Autodesk Fusion 360 part; units mm, degrees
(part 3 of 6)
  constraint coincident L336.end L337.start
  constraint perpendicular L693 L694
  constraint parallel L693 L695
  constraint parallel L694 L696
  constraint coincident L473.end L474.start
  constraint perpendicular L473 L693
  constraint coincident L504.end L505.start
  constraint perpendicular L697 L698
  constraint parallel L697 L699
  constraint parallel L698 L700
  constraint perpendicular L701 L702
  constraint parallel L701 L703
  constraint parallel L702 L704
  constraint coincident L458.end L459.start
  constraint perpendicular L458 L701
  constraint coincident L474.end L475.start
  constraint perpendicular L705 L706
  constraint parallel L705 L707
  constraint parallel L706 L708
  constraint perpendicular L709 L710
  constraint parallel L709 L711
  constraint parallel L710 L712
  constraint coincident L429.end L430.start
  constraint perpendicular L429 L709
  constraint coincident L440.start L459.end
  constraint perpendicular L713 L714
  constraint parallel L713 L715
  constraint parallel L714 L716
  constraint perpendicular L717 L718
  constraint parallel L717 L719
  constraint parallel L718 L720
  constraint coincident L385.end L386.start
  constraint perpendicular L385 L717
  constraint coincident L430.end L431.start
  constraint perpendicular L721 L722
  constraint parallel L721 L723
  constraint parallel L722 L724
  constraint coincident L356.end L357.start
  constraint perpendicular L357 L721
  constraint coincident L420.start L439.end
  constraint perpendicular L725 L726
  constraint parallel L725 L727
  constraint parallel L726 L728
  constraint coincident L386.end L387.start
  constraint perpendicular L387 L725
  constraint coincident L410.end L411.start
  constraint perpendicular L729 L730
  constraint parallel L729 L731
  constraint parallel L730 L732
  constraint coincident L401.end L402.start
  constraint perpendicular L402 L729
  constraint coincident L355.end L356.start
  constraint perpendicular L733 L734
  constraint parallel L733 L735
  constraint parallel L734 L736
  constraint coincident L484.end L485.start
  constraint perpendicular L485 L733
  constraint coincident L400.end L401.start
  constraint perpendicular L737 L738
  constraint parallel L737 L739
  constraint parallel L738 L740
  constraint coincident L493.end L494.start
  constraint perpendicular L493 L737
  constraint coincident L411.end L412.start
  constraint perpendicular L741 L742
  constraint parallel L741 L743
  constraint parallel L742 L744
  constraint coincident L326.end L327.start
  constraint perpendicular L326 L741
  constraint coincident L494.end L495.start
  constraint perpendicular L745 L746
  constraint parallel L745 L747
  constraint parallel L746 L748
  constraint coincident L337.end L338.start
  constraint perpendicular L338 L745
  constraint coincident L483.end L484.start
  constraint perpendicular L749 L750
  constraint parallel L749 L751
  constraint parallel L750 L752
  constraint coincident L127.end L128.start
  constraint perpendicular L127 L749
  constraint coincident L586.end L587.start
  constraint perpendicular L753 L754
  constraint parallel L753 L755
  constraint parallel L754 L756
  constraint coincident L595.end L596.start
  constraint perpendicular L595 L753
  constraint coincident L138.end L139.start
  constraint perpendicular L757 L758
  constraint parallel L757 L759
  constraint parallel L758 L760
  constraint coincident L294.end L295.start
  constraint perpendicular L295 L757
  constraint coincident L81.end L82.start
  constraint perpendicular L761 L762
  constraint parallel L761 L763
  constraint parallel L762 L764
  constraint coincident L92.end L93.start
  constraint perpendicular L93 L761
  constraint coincident L283.end L284.start
  constraint perpendicular L765 L766
  constraint parallel L765 L767
  constraint parallel L766 L768
  constraint coincident L197.end L198.start
  constraint perpendicular L198 L765
  constraint coincident L91.end L92.start
  constraint perpendicular L769 L770
  constraint parallel L769 L771
  constraint parallel L770 L772
  constraint perpendicular L773 L774
  constraint parallel L773 L775
  constraint parallel L774 L776
  constraint coincident L545.end L546.start
  constraint perpendicular L546 L773
  constraint coincident L571.end L572.start
  constraint perpendicular L777 L778
  constraint parallel L777 L779
  constraint parallel L778 L780
  constraint perpendicular L781 L782
  constraint parallel L781 L783
  constraint parallel L782 L784
  constraint coincident L151.end L152.start
  constraint perpendicular L152 L781
  constraint coincident L162.end L163.start
  constraint perpendicular L785 L786
  constraint parallel L785 L787
  constraint parallel L786 L788
  constraint perpendicular L789 L790
  constraint parallel L789 L791
  constraint parallel L790 L792
  constraint coincident L28.end L29.start
  constraint perpendicular L28 L789
  constraint coincident L536.end L537.start
  constraint perpendicular L793 L794
  constraint parallel L793 L795
  constraint parallel L794 L796
  constraint perpendicular L797 L798
  constraint parallel L797 L799
  constraint parallel L798 L800
  constraint coincident L232.end L233.start
  constraint perpendicular L233 L797
  constraint coincident L213.end L214.start
  constraint perpendicular L801 L802
  constraint parallel L801 L803
  constraint parallel L802 L804
  constraint perpendicular L805 L806
  constraint parallel L805 L807
  constraint parallel L806 L808
  constraint coincident L70.end L71.start
  constraint perpendicular L70 L805
  constraint coincident L51.end L52.start
  constraint perpendicular L809 L810
  constraint parallel L809 L811
  constraint parallel L810 L812
  constraint perpendicular L813 L814
  constraint parallel L813 L815
  constraint parallel L814 L816
  constraint coincident L277.end L278.start
  constraint perpendicular L278 L813
  constraint coincident L240.start L259.end
  constraint perpendicular L817 L818
  constraint parallel L817 L819
  constraint parallel L818 L820
  constraint perpendicular L821 L822
  constraint parallel L821 L823
  constraint parallel L822 L824
  constraint coincident L107.end L108.start
  constraint perpendicular L107 L821
  constraint coincident L17.end L18.start
  constraint perpendicular L825 L826
  constraint parallel L825 L827
  constraint parallel L826 L828
  constraint perpendicular L829 L830
  constraint parallel L829 L831
  constraint parallel L830 L832
  constraint coincident L284.end L285.start
  constraint perpendicular L285 L829
  constraint coincident L317.end L318.start
  constraint perpendicular L833 L834
  constraint parallel L833 L835
  constraint parallel L834 L836
  measures "d21" distance of L503.end L687.end
  measures "d22" distance of L336.end L691.end
  measures "d23" distance of L586.end L751.end
  measures "d24" distance of L138.end L755.end
  measures "d25" distance of L81.end L759.end
  measures "d26" distance of L283.end L763.end
extrude "Extrude4" cut sketch "Sketch3" against normal blind 20 contours L17 L753 L755 L820 L824 L826 | L108 L753 L755 L822 L828 L834 | L71 L753 L755 L806 L812 L818 | L7 L749 L751 L820 L826 | L138 L753 L755 L756 L836 | L118 L749 L751 L828 L834 | L51 L753 L755 L804 L808 L810 | L61 L749 L751 L812 L818 | L267 L757 L759 L820 L826 | L128 L749 L750 L751 L836 | L308 L757 L759 L828 L834 | L29 L753 L755 L790 L796 L802 | L41 L749 L751 L804 L810 | L250 L757 L759 L812 L818 | L294 L757 L758 L759 L836 | L536 L753 L755 L788 L792 L794 | L39 L749 L751 L796 L802 | L222 L757 L759 L804 L810 | L572 L753 L755 L776 L778 L786 | L526 L749 L751 L788 L794 | L204 L757 L759 L796 L802 | L277 L761 L763 L814 L820 L826 | L318 L761 L763 L828 L832 L834 | L545 L753 L755 L772 L774 L780 | L562 L749 L751 L778 L786 | L141 L757 L759 L788 L794 | L240 L761 L763 L812 L816 L818 | L284 L761 L763 L764 L830 L836 | L596 L753 L754 L755 L770 | L555 L749 L751 L772 L780 | L173 L757 L759 L778 L786 | L232 L761 L763 L798 L804 L810 | L586 L749 L751 L752 L770 | L187 L757 L759 L772 L780 | L214 L761 L763 L796 L800 L802 | L82 L757 L759 L760 L770 | L151 L761 L763 L782 L788 L794 | L163 L761 L763 L778 L784 L786 | L197 L761 L763 L766 L772 L780 | L92 L761 L762 L763 L768 L770 | L337 L689 L691 L692 L746 | L484 L689 L691 L734 L748 | L401 L689 L691 L730 L736 | L327 L685 L686 L687 L742 | L494 L685 L687 L738 L744 | L356 L689 L691 L722 L732 | L411 L685 L687 L728 L740 | L420 L689 L691 L714 L724 | L386 L685 L687 L718 L726 | L449 L689 L691 L708 L716 | L430 L685 L687 L710 L714 L720 | L464 L689 L691 L698 L706 | L459 L685 L687 L702 L708 L712 L716 | L514 L689 L690 L691 L700 | L474 L685 L687 L694 L698 L704 L706 | L504 L685 L687 L688 L696 L700
extrude "Extrude6" add sketch "Sketch3" against normal blind 1 contours L17 L753 L755 L820 L824 L826 | L108 L753 L755 L822 L828 L834 | L71 L753 L755 L806 L812 L818 | L7 L749 L751 L820 L826 | L138 L753 L755 L756 L836 | L118 L749 L751 L828 L834 | L51 L753 L755 L804 L808 L810 | L61 L749 L751 L812 L818 | L267 L757 L759 L820 L826 | L128 L749 L750 L751 L836 | L308 L757 L759 L828 L834 | L29 L753 L755 L790 L796 L802 | L41 L749 L751 L804 L810 | L250 L757 L759 L812 L818 | L294 L757 L758 L759 L836 | L536 L753 L755 L788 L792 L794 | L39 L749 L751 L796 L802 | L222 L757 L759 L804 L810 | L572 L753 L755 L776 L778 L786 | L526 L749 L751 L788 L794 | L204 L757 L759 L796 L802 | L277 L761 L763 L814 L820 L826 | L318 L761 L763 L828 L832 L834 | L545 L753 L755 L772 L774 L780 | L562 L749 L751 L778 L786 | L141 L757 L759 L788 L794 | L240 L761 L763 L812 L816 L818 | L284 L761 L763 L764 L830 L836 | L596 L753 L754 L755 L770 | L555 L749 L751 L772 L780 | L173 L757 L759 L778 L786 | L232 L761 L763 L798 L804 L810 | L586 L749 L751 L752 L770 | L187 L757 L759 L772 L780 | L214 L761 L763 L796 L800 L802 | L82 L757 L759 L760 L770 | L151 L761 L763 L782 L788 L794 | L163 L761 L763 L778 L784 L786 | L197 L761 L763 L766 L772 L780 | L92 L761 L762 L763 L768 L770 | L337 L689 L691 L692 L746 | L484 L689 L691 L734 L748 | L401 L689 L691 L730 L736 | L327 L685 L686 L687 L742 | L494 L685 L687 L738 L744 | L356 L689 L691 L722 L732 | L411 L685 L687 L728 L740 | L420 L689 L691 L714 L724 | L386 L685 L687 L718 L726 | L449 L689 L691 L708 L716 | L430 L685 L687 L710 L714 L720 | L464 L689 L691 L698 L706 | L459 L685 L687 L702 L708 L712 L716 | L514 L689 L690 L691 L700 | L474 L685 L687 L694 L698 L704 L706 | L504 L685 L687 L688 L696 L700
sketch "Sketch4" plane through (0, -4, 0) normal (0, -1, 0) x (1, 0, 0)
  line L0 (39.9203, -25.9319) -> (39.9203, -22.8327)
  line L1 (39.9203, -22.8327) -> (40.7211, -22.8327)
  line L2 (40.7211, -22.8327) -> (40.7211, -20.8323)
  line L3 (54.7204, -20.8323) -> (54.7204, -22.8327)
  line L4 (54.7204, -22.8327) -> (55.5212, -22.8327)
  line L5 (55.5212, -22.8327) -> (55.5212, -25.9319)
  line L6 (55.5212, -25.9319) -> (54.7204, -25.9319)
  line L7 (54.7204, -25.9319) -> (54.7204, -31.7321)
  line L8 (54.7204, -31.7321) -> (55.5212, -31.7321)
  line L9 (55.5212, -31.7321) -> (55.5212, -34.8327)
  line L10 (55.5212, -34.8327) -> (54.7204, -34.8327)
  line L11 (54.7204, -34.8327) -> (54.7204, -36.8316)
  line L12 (40.7211, -36.8316) -> (40.7211, -34.8327)
  line L13 (40.7211, -34.8327) -> (39.9203, -34.8327)
  line L14 (39.9203, -34.8327) -> (39.9203, -31.7321)
  line L15 (39.9203, -31.7321) -> (40.7211, -31.7321)
  line L16 (40.7211, -31.7321) -> (40.7211, -25.9319)
  line L17 (40.7211, -25.9319) -> (39.9203, -25.9319)
  line L18 (111.869, -34.8327) -> (111.869, -36.8316)
  line L19 (97.8697, -36.8316) -> (97.8697, -34.8327)
  line L20 (97.8697, -34.8327) -> (97.0703, -34.8327)
  line L21 (97.0703, -34.8327) -> (97.0703, -31.7321)
  line L22 (97.0703, -31.7321) -> (97.8697, -31.7321)
  line L23 (97.8697, -31.7321) -> (97.8697, -25.9319)
  line L24 (97.8697, -25.9319) -> (97.0703, -25.9319)
  line L25 (97.0703, -25.9319) -> (97.0703, -22.8327)
  line L26 (97.0703, -22.8327) -> (97.8697, -22.8327)
  line L27 (97.8697, -22.8327) -> (97.8697, -20.8323)
  line L28 (111.869, -20.8323) -> (111.869, -22.8327)
  line L29 (111.869, -22.8327) -> (112.67, -22.8327)
  line L30 (112.67, -22.8327) -> (112.67, -25.9319)
  line L31 (112.67, -25.9319) -> (111.869, -25.9319)
  line L32 (111.869, -25.9319) -> (111.869, -31.7321)
  line L33 (111.869, -31.7321) -> (112.67, -31.7321)
  line L34 (112.67, -31.7321) -> (112.67, -34.8327)
  line L35 (112.67, -34.8327) -> (111.869, -34.8327)
  line L36 (78.8211, -36.8316) -> (78.8211, -34.8327)
  line L37 (78.8211, -34.8327) -> (78.0203, -34.8327)
  line L38 (78.0203, -34.8327) -> (78.0203, -31.7321)
  line L39 (78.0203, -31.7321) -> (78.8211, -31.7321)
  line L40 (78.8211, -31.7321) -> (78.8211, -25.9319)
  line L41 (78.8211, -25.9319) -> (78.0203, -25.9319)
  line L42 (78.0203, -25.9319) -> (78.0203, -22.8327)
  line L43 (78.0203, -22.8327) -> (78.8211, -22.8327)
  line L44 (78.8211, -22.8327) -> (78.8211, -20.8323)
  line L45 (92.8204, -20.8323) -> (92.8204, -22.8327)
  line L46 (92.8204, -22.8327) -> (93.6198, -22.8327)
  line L47 (93.6198, -22.8327) -> (93.6198, -25.9319)
  line L48 (93.6198, -25.9319) -> (92.8204, -25.9319)
  line L49 (92.8204, -25.9319) -> (92.8204, -31.7321)
  line L50 (92.8204, -31.7321) -> (93.6198, -31.7321)
  line L51 (93.6198, -31.7321) -> (93.6198, -34.8327)
  line L52 (93.6198, -34.8327) -> (92.8204, -34.8327)
  line L53 (92.8204, -34.8327) -> (92.8204, -36.8316)
  line L54 (59.7711, -36.8316) -> (59.7711, -34.8327)
  line L55 (59.7711, -34.8327) -> (58.9703, -34.8327)
  line L56 (58.9703, -34.8327) -> (58.9703, -31.7321)
  line L57 (58.9703, -31.7321) -> (59.7711, -31.7321)
  line L58 (59.7711, -31.7321) -> (59.7711, -25.9319)
  line L59 (59.7711, -25.9319) -> (58.9703, -25.9319)
  line L60 (58.9703, -25.9319) -> (58.9703, -22.8327)
  line L61 (58.9703, -22.8327) -> (59.7711, -22.8327)
  line L62 (59.7711, -22.8327) -> (59.7711, -20.8323)
  line L63 (73.7704, -20.8323) -> (73.7704, -22.8327)
  line L64 (73.7704, -22.8327) -> (74.5712, -22.8327)
  line L65 (74.5712, -22.8327) -> (74.5712, -25.9319)
  line L66 (74.5712, -25.9319) -> (73.7704, -25.9319)
  line L67 (73.7704, -25.9319) -> (73.7704, -31.7321)
  line L68 (73.7704, -31.7321) -> (74.5712, -31.7321)
  line L69 (74.5712, -31.7321) -> (74.5712, -34.8327)
  line L70 (74.5712, -34.8327) -> (73.7704, -34.8327)
  line L71 (73.7704, -34.8327) -> (73.7704, -36.8316)
  line L72 (188.07, -41.8828) -> (188.871, -41.8828)
  line L73 (188.871, -41.8828) -> (188.871, -44.982)
  line L74 (188.871, -44.982) -> (188.07, -44.982)
  line L75 (188.07, -44.982) -> (188.07, -50.782)
  line L76 (188.07, -50.782) -> (188.871, -50.782)
  line L77 (188.871, -50.782) -> (188.871, -53.8826)
  line L78 (188.871, -53.8826) -> (188.07, -53.8826)
  line L79 (188.07, -53.8826) -> (188.07, -55.8816)
  line L80 (174.071, -55.8816) -> (174.071, -53.8826)
  line L81 (174.071, -53.8826) -> (173.27, -53.8826)
  line L82 (173.27, -53.8826) -> (173.27, -50.782)
  line L83 (173.27, -50.782) -> (174.071, -50.782)
  line L84 (174.071, -50.782) -> (174.071, -44.982)
  line L85 (174.071, -44.982) -> (173.27, -44.982)
  line L86 (173.27, -44.982) -> (173.27, -41.8828)
  line L87 (173.27, -41.8828) -> (174.071, -41.8828)
  line L88 (174.071, -41.8828) -> (174.071, -39.8824)
  line L89 (188.07, -39.8824) -> (188.07, -41.8828)
  line L90 (36.4712, -34.8327) -> (35.6704, -34.8327)
  line L91 (35.6704, -34.8327) -> (35.6704, -36.8316)
  line L92 (21.671, -36.8316) -> (21.671, -34.8327)
  line L93 (21.671, -34.8327) -> (20.8704, -34.8327)
  line L94 (20.8704, -34.8327) -> (20.8704, -31.7321)
  line L95 (20.8704, -31.7321) -> (21.671, -31.7321)
  line L96 (21.671, -31.7321) -> (21.671, -25.9319)
  line L97 (21.671, -25.9319) -> (20.8704, -25.9319)
  line L98 (20.8704, -25.9319) -> (20.8704, -22.8327)
  line L99 (20.8704, -22.8327) -> (21.671, -22.8327)
  line L100 (21.671, -22.8327) -> (21.671, -20.8323)
  line L101 (35.6704, -20.8323) -> (35.6704, -22.8327)
  line L102 (35.6704, -22.8327) -> (36.4712, -22.8327)
  line L103 (36.4712, -22.8327) -> (36.4712, -25.9319)
  line L104 (36.4712, -25.9319) -> (35.6704, -25.9319)
  line L105 (35.6704, -25.9319) -> (35.6704, -31.7321)
  line L106 (35.6704, -31.7321) -> (36.4712, -31.7321)
  line L107 (36.4712, -31.7321) -> (36.4712, -34.8327)
  line L108 (1.8204, -22.8327) -> (2.621, -22.8327)
  line L109 (2.621, -22.8327) -> (2.621, -20.8323)
  line L110 (16.6205, -20.8323) -> (16.6205, -22.8327)
  line L111 (16.6205, -22.8327) -> (17.4212, -22.8327)
  line L112 (17.4212, -22.8327) -> (17.4212, -25.9319)
  line L113 (17.4212, -25.9319) -> (16.6205, -25.9319)
  line L114 (16.6205, -25.9319) -> (16.6205, -31.7321)
  line L115 (16.6205, -31.7321) -> (17.4212, -31.7321)
  line L116 (17.4212, -31.7321) -> (17.4212, -34.8327)
  line L117 (17.4212, -34.8327) -> (16.6205, -34.8327)
  line L118 (16.6205, -34.8327) -> (16.6205, -36.8316)
  line L119 (2.621, -36.8316) -> (2.621, -34.8327)
  line L120 (2.621, -34.8327) -> (1.8204, -34.8327)
  line L121 (1.8204, -34.8327) -> (1.8204, -31.7321)
  line L122 (1.8204, -31.7321) -> (2.621, -31.7321)
  line L123 (2.621, -31.7321) -> (2.621, -25.9319)
  line L124 (2.621, -25.9319) -> (1.8204, -25.9319)
  line L125 (1.8204, -25.9319) -> (1.8204, -22.8327)
  line L126 (130.92, -39.8824) -> (130.92, -41.8828)
  line L127 (130.92, -41.8828) -> (131.721, -41.8828)
  line L128 (131.721, -41.8828) -> (131.721, -44.982)
  line L129 (131.721, -44.982) -> (130.92, -44.982)
  line L130 (130.92, -44.982) -> (130.92, -50.782)
  line L131 (130.92, -50.782) -> (131.721, -50.782)
  line L132 (131.721, -50.782) -> (131.721, -53.8826)
  line L133 (131.721, -53.8826) -> (130.92, -53.8826)
  line L134 (130.92, -53.8826) -> (130.92, -55.8816)
  line L135 (116.92, -55.8816) -> (116.92, -53.8826)
  line L136 (116.92, -53.8826) -> (116.119, -53.8826)
  line L137 (116.119, -53.8826) -> (116.119, -50.782)
  line L138 (116.119, -50.782) -> (116.92, -50.782)
  line L139 (116.92, -50.782) -> (116.92, -44.982)
  line L140 (116.92, -44.982) -> (116.119, -44.982)
  line L141 (116.119, -44.982) -> (116.119, -41.8828)
  line L142 (116.119, -41.8828) -> (116.92, -41.8828)
  line L143 (116.92, -41.8828) -> (116.92, -39.8824)
  line L144 (135.17, -53.8826) -> (135.17, -50.782)
  line L145 (135.17, -50.782) -> (135.971, -50.782)
  line L146 (135.971, -50.782) -> (135.971, -44.982)
  line L147 (135.971, -44.982) -> (135.17, -44.982)
  line L148 (135.17, -44.982) -> (135.17, -41.8828)
  line L149 (135.17, -41.8828) -> (135.971, -41.8828)
  line L150 (135.971, -41.8828) -> (135.971, -39.8824)
  line L151 (149.97, -39.8824) -> (149.97, -41.8828)
  line L152 (149.97, -41.8828) -> (150.771, -41.8828)
  line L153 (150.771, -41.8828) -> (150.771, -44.982)
  line L154 (150.771, -44.982) -> (149.97, -44.982)
  line L155 (149.97, -44.982) -> (149.97, -50.782)
  line L156 (149.97, -50.782) -> (150.771, -50.782)
  line L157 (150.771, -50.782) -> (150.771, -53.8826)
  line L158 (150.771, -53.8826) -> (149.97, -53.8826)
  line L159 (149.97, -53.8826) -> (149.97, -55.8816)
  line L160 (135.971, -55.8816) -> (135.971, -53.8826)
  line L161 (135.971, -53.8826) -> (135.17, -53.8826)
  line L162 (169.821, -50.782) -> (169.821, -53.8826)
  line L163 (169.821, -53.8826) -> (169.02, -53.8826)
  line L164 (169.02, -53.8826) -> (169.02, -55.8816)
  line L165 (155.021, -55.8816) -> (155.021, -53.8826)
  line L166 (155.021, -53.8826) -> (154.22, -53.8826)
  line L167 (154.22, -53.8826) -> (154.22, -50.782)
  line L168 (154.22, -50.782) -> (155.021, -50.782)
  line L169 (155.021, -50.782) -> (155.021, -44.982)
  line L170 (155.021, -44.982) -> (154.22, -44.982)
  line L171 (154.22, -44.982) -> (154.22, -41.8828)
  line L172 (154.22, -41.8828) -> (155.021, -41.8828)
  line L173 (155.021, -41.8828) -> (155.021, -39.8824)
  line L174 (169.02, -39.8824) -> (169.02, -41.8828)
  line L175 (169.02, -41.8828) -> (169.821, -41.8828)
  line L176 (169.821, -41.8828) -> (169.821, -44.982)
  line L177 (169.821, -44.982) -> (169.02, -44.982)
  line L178 (169.02, -44.982) -> (169.02, -50.782)
  line L179 (169.02, -50.782) -> (169.821, -50.782)
  line L180 (112.67, -44.982) -> (111.869, -44.982)
  line L181 (111.869, -44.982) -> (111.869, -50.782)
  line L182 (111.869, -50.782) -> (112.67, -50.782)
  line L183 (112.67, -50.782) -> (112.67, -53.8826)
  line L184 (112.67, -53.8826) -> (111.869, -53.8826)
  line L185 (111.869, -53.8826) -> (111.869, -55.8816)
  line L186 (97.8697, -55.8816) -> (97.8697, -53.8826)
  line L187 (97.8697, -53.8826) -> (97.0703, -53.8826)
  line L188 (97.0703, -53.8826) -> (97.0703, -50.782)
  line L189 (97.0703, -50.782) -> (97.8697, -50.782)
  line L190 (97.8697, -50.782) -> (97.8697, -44.982)
  line L191 (97.8697, -44.982) -> (97.0703, -44.982)
  line L192 (97.0703, -44.982) -> (97.0703, -41.8828)
  line L193 (97.0703, -41.8828) -> (97.8697, -41.8828)
  line L194 (97.8697, -41.8828) -> (97.8697, -39.8824)
  line L195 (111.869, -39.8824) -> (111.869, -41.8828)
  line L196 (111.869, -41.8828) -> (112.67, -41.8828)
  line L197 (112.67, -41.8828) -> (112.67, -44.982)
  line L198 (92.8204, -41.8828) -> (93.6198, -41.8828)
  line L199 (93.6198, -41.8828) -> (93.6198, -44.982)
  line L200 (93.6198, -44.982) -> (92.8204, -44.982)
  line L201 (92.8204, -44.982) -> (92.8204, -50.782)
  line L202 (92.8204, -50.782) -> (93.6198, -50.782)
  line L203 (93.6198, -50.782) -> (93.6198, -53.8826)
  line L204 (93.6198, -53.8826) -> (92.8204, -53.8826)
  line L205 (92.8204, -53.8826) -> (92.8204, -55.8816)
  line L206 (78.8211, -55.8816) -> (78.8211, -53.8826)
  line L207 (78.8211, -53.8826) -> (78.0203, -53.8826)
  line L208 (78.0203, -53.8826) -> (78.0203, -50.782)
  line L209 (78.0203, -50.782) -> (78.8211, -50.782)
  line L210 (78.8211, -50.782) -> (78.8211, -44.982)
  line L211 (78.8211, -44.982) -> (78.0203, -44.982)
  line L212 (78.0203, -44.982) -> (78.0203, -41.8828)
  line L213 (78.0203, -41.8828) -> (78.8211, -41.8828)
  line L214 (78.8211, -41.8828) -> (78.8211, -39.8824)
  line L215 (92.8204, -39.8824) -> (92.8204, -41.8828)
  line L216 (59.7711, -55.8816) -> (59.7711, -53.8826)
  line L217 (59.7711, -53.8826) -> (58.9703, -53.8826)
  line L218 (58.9703, -53.8826) -> (58.9703, -50.782)
  line L219 (58.9703, -50.782) -> (59.7711, -50.782)
  line L220 (59.7711, -50.782) -> (59.7711, -44.982)
  line L221 (59.7711, -44.982) -> (58.9703, -44.982)
  line L222 (58.9703, -44.982) -> (58.9703, -41.8828)
  line L223 (58.9703, -41.8828) -> (59.7711, -41.8828)
  line L224 (59.7711, -41.8828) -> (59.7711, -39.8824)
  line L225 (73.7704, -39.8824) -> (73.7704, -41.8828)
  line L226 (73.7704, -41.8828) -> (74.5712, -41.8828)
  line L227 (74.5712, -41.8828) -> (74.5712, -44.982)
  line L228 (74.5712, -44.982) -> (73.7704, -44.982)
  line L229 (73.7704, -44.982) -> (73.7704, -50.782)
  line L230 (73.7704, -50.782) -> (74.5712, -50.782)
  line L231 (74.5712, -50.782) -> (74.5712, -53.8826)
  line L232 (74.5712, -53.8826) -> (73.7704, -53.8826)
  line L233 (73.7704, -53.8826) -> (73.7704, -55.8816)
  line L234 (55.5212, -50.782) -> (55.5212, -53.8826)
  line L235 (55.5212, -53.8826) -> (54.7204, -53.8826)
  line L236 (54.7204, -53.8826) -> (54.7204, -55.8816)
  line L237 (40.7211, -55.8816) -> (40.7211, -53.8826)
  line L238 (40.7211, -53.8826) -> (39.9203, -53.8826)
  line L239 (39.9203, -53.8826) -> (39.9203, -50.782)
  line L240 (39.9203, -50.782) -> (40.7211, -50.782)
  line L241 (40.7211, -50.782) -> (40.7211, -44.982)
  line L242 (40.7211, -44.982) -> (39.9203, -44.982)
  line L243 (39.9203, -44.982) -> (39.9203, -41.8828)
  line L244 (39.9203, -41.8828) -> (40.7211, -41.8828)
  line L245 (40.7211, -41.8828) -> (40.7211, -39.8824)
  line L246 (54.7204, -39.8824) -> (54.7204, -41.8828)
  line L247 (54.7204, -41.8828) -> (55.5212, -41.8828)
  line L248 (55.5212, -41.8828) -> (55.5212, -44.982)
  line L249 (55.5212, -44.982) -> (54.7204, -44.982)
  line L250 (54.7204, -44.982) -> (54.7204, -50.782)
  line L251 (54.7204, -50.782) -> (55.5212, -50.782)
  line L252 (1.8204, -50.782) -> (2.621, -50.782)
  line L253 (2.621, -50.782) -> (2.621, -44.982)
  line L254 (2.621, -44.982) -> (1.8204, -44.982)
  line L255 (1.8204, -44.982) -> (1.8204, -41.8828)
  line L256 (1.8204, -41.8828) -> (2.621, -41.8828)
  line L257 (2.621, -41.8828) -> (2.621, -39.8824)
  line L258 (16.6205, -39.8824) -> (16.6205, -41.8828)
  line L259 (16.6205, -41.8828) -> (17.4212, -41.8828)
  line L260 (17.4212, -41.8828) -> (17.4212, -44.982)
  line L261 (17.4212, -44.982) -> (16.6205, -44.982)
  line L262 (16.6205, -44.982) -> (16.6205, -50.782)
  line L263 (16.6205, -50.782) -> (17.4212, -50.782)
  line L264 (17.4212, -50.782) -> (17.4212, -53.8826)
  line L265 (17.4212, -53.8826) -> (16.6205, -53.8826)
  line L266 (16.6205, -53.8826) -> (16.6205, -55.8816)
  line L267 (2.621, -55.8816) -> (2.621, -53.8826)
  line L268 (2.621, -53.8826) -> (1.8204, -53.8826)
  line L269 (1.8204, -53.8826) -> (1.8204, -50.782)
  line L270 (36.4712, -53.8826) -> (35.6704, -53.8826)
  line L271 (35.6704, -53.8826) -> (35.6704, -55.8816)
  line L272 (21.671, -55.8816) -> (21.671, -53.8826)
  line L273 (21.671, -53.8826) -> (20.8704, -53.8826)
  line L274 (20.8704, -53.8826) -> (20.8704, -50.782)
  line L275 (20.8704, -50.782) -> (21.671, -50.782)
  line L276 (21.671, -50.782) -> (21.671, -44.982)
  line L277 (21.671, -44.982) -> (20.8704, -44.982)
  line L278 (20.8704, -44.982) -> (20.8704, -41.8828)
  line L279 (20.8704, -41.8828) -> (21.671, -41.8828)
  line L280 (21.671, -41.8828) -> (21.671, -39.8824)
  line L281 (35.6704, -39.8824) -> (35.6704, -41.8828)
  line L282 (35.6704, -41.8828) -> (36.4712, -41.8828)
  line L283 (36.4712, -41.8828) -> (36.4712, -44.982)
  line L284 (36.4712, -44.982) -> (35.6704, -44.982)
  line L285 (35.6704, -44.982) -> (35.6704, -50.782)
  line L286 (35.6704, -50.782) -> (36.4712, -50.782)
  line L287 (36.4712, -50.782) -> (36.4712, -53.8826)
  line L288 (163.745, -6.8819) -> (163.745, -3.7827)
  line L289 (163.745, -3.7827) -> (164.546, -3.7827)
  line L290 (164.546, -3.7827) -> (164.546, -1.7823)
  line L291 (178.545, -1.7823) -> (178.545, -3.7827)
  line L292 (178.545, -3.7827) -> (179.346, -3.7827)
  line L293 (179.346, -3.7827) -> (179.346, -6.8819)
  line L294 (179.346, -6.8819) -> (178.545, -6.8819)
  line L295 (178.545, -6.8819) -> (178.545, -12.6821)
  line L296 (178.545, -12.6821) -> (179.346, -12.6821)
  line L297 (179.346, -12.6821) -> (179.346, -15.7827)
  line L298 (179.346, -15.7827) -> (178.545, -15.7827)
  line L299 (178.545, -15.7827) -> (178.545, -17.7817)
  line L300 (164.546, -17.7817) -> (164.546, -15.7827)
  line L301 (164.546, -15.7827) -> (163.745, -15.7827)
  line L302 (163.745, -15.7827) -> (163.745, -12.6821)
  line L303 (163.745, -12.6821) -> (164.546, -12.6821)
  line L304 (164.546, -12.6821) -> (164.546, -6.8819)
  line L305 (164.546, -6.8819) -> (163.745, -6.8819)
  line L306 (120.971, -12.0826) -> (120.146, -12.0826)
  line L307 (120.146, -12.0826) -> (120.146, -15.3128)
  line L308 (120.146, -15.3128) -> (118.42, -15.3128)
  line L309 (118.42, -15.3128) -> (118.42, -16.2319)
  line L310 (118.42, -16.2319) -> (115.12, -16.2319)
  line L311 (115.12, -16.2319) -> (115.12, -15.3128)
  line L312 (115.12, -15.3128) -> (113.396, -15.3128)
  line L313 (113.396, -15.3128) -> (113.396, -12.0826)
  line L314 (113.396, -12.0826) -> (111.87, -12.0826)
  line L315 (111.87, -12.0826) -> (111.87, -12.6821)
  line L316 (111.87, -12.6821) -> (112.671, -12.6821)
  line L317 (112.671, -12.6821) -> (112.671, -15.7827)
  line L318 (112.671, -15.7827) -> (111.87, -15.7827)
  line L319 (111.87, -15.7827) -> (111.87, -17.7817)
  line L320 (97.8711, -17.7817) -> (97.8711, -15.7827)
  line L321 (97.8711, -15.7827) -> (97.0703, -15.7827)
  line L322 (97.0703, -15.7827) -> (97.0703, -12.6821)
  line L323 (97.0703, -12.6821) -> (97.8711, -12.6821)
  line L324 (97.8711, -12.6821) -> (97.8711, -12.0826)
  line L325 (97.8711, -12.0826) -> (96.3454, -12.0826)
  line L326 (96.3454, -12.0826) -> (96.3454, -15.3128)
  line L327 (96.3454, -15.3128) -> (94.6203, -15.3128)
  line L328 (94.6203, -15.3128) -> (94.6203, -16.2319)
  line L329 (94.6203, -16.2319) -> (91.3197, -16.2319)
  line L330 (91.3197, -16.2319) -> (91.3197, -15.3128)
  line L331 (91.3197, -15.3128) -> (89.596, -15.3128)
  line L332 (89.596, -15.3128) -> (89.596, -12.0826)
  line L333 (89.596, -12.0826) -> (88.7705, -12.0826)
  line L334 (88.7705, -12.0826) -> (88.7705, -9.2825)
  line L335 (88.7705, -9.2825) -> (89.596, -9.2825)
  line L336 (89.596, -9.2825) -> (89.596, -3.0138)
  line L337 (89.596, -3.0138) -> (91.3197, -3.0138)
  line L338 (91.3197, -3.0138) -> (91.3197, -2.0326)
  line L339 (91.3197, -2.0326) -> (94.6203, -2.0326)
  line L340 (94.6203, -2.0326) -> (94.6203, -3.0138)
  line L341 (94.6203, -3.0138) -> (96.3454, -3.0138)
  line L342 (96.3454, -3.0138) -> (96.3454, -7.4827)
  line L343 (96.3454, -7.4827) -> (97.8711, -7.4827)
  line L344 (97.8711, -7.4827) -> (97.8711, -6.8819)
  line L345 (97.8711, -6.8819) -> (97.0703, -6.8819)
  line L346 (97.0703, -6.8819) -> (97.0703, -3.7827)
  line L347 (97.0703, -3.7827) -> (97.8711, -3.7827)
  line L348 (97.8711, -3.7827) -> (97.8711, -1.7823)
  line L349 (111.87, -1.7823) -> (111.87, -3.7827)
  line L350 (111.87, -3.7827) -> (112.671, -3.7827)
  line L351 (112.671, -3.7827) -> (112.671, -6.8819)
  line L352 (112.671, -6.8819) -> (111.87, -6.8819)
  line L353 (111.87, -6.8819) -> (111.87, -7.4827)
  line L354 (111.87, -7.4827) -> (113.396, -7.4827)
  line L355 (113.396, -7.4827) -> (113.396, -3.0138)
  line L356 (113.396, -3.0138) -> (115.12, -3.0138)
  line L357 (115.12, -3.0138) -> (115.12, -2.0326)
  line L358 (115.12, -2.0326) -> (118.42, -2.0326)
  line L359 (118.42, -2.0326) -> (118.42, -3.0138)
  line L360 (118.42, -3.0138) -> (120.146, -3.0138)
  line L361 (120.146, -3.0138) -> (120.146, -9.2825)
  line L362 (120.146, -9.2825) -> (120.971, -9.2825)
  line L363 (120.971, -9.2825) -> (120.971, -12.0826)
  line L364 (140.445, -1.7823) -> (140.445, -3.7827)
  line L365 (140.445, -3.7827) -> (141.246, -3.7827)
  line L366 (141.246, -3.7827) -> (141.246, -6.8819)
  line L367 (141.246, -6.8819) -> (140.445, -6.8819)
  line L368 (140.445, -6.8819) -> (140.445, -12.6821)
  line L369 (140.445, -12.6821) -> (141.246, -12.6821)
  line L370 (141.246, -12.6821) -> (141.246, -15.7827)
  line L371 (141.246, -15.7827) -> (140.445, -15.7827)
  line L372 (140.445, -15.7827) -> (140.445, -17.7817)
  line L373 (126.446, -17.7817) -> (126.446, -15.7827)
  line L374 (126.446, -15.7827) -> (125.645, -15.7827)
  line L375 (125.645, -15.7827) -> (125.645, -12.6821)
  line L376 (125.645, -12.6821) -> (126.446, -12.6821)
  line L377 (126.446, -12.6821) -> (126.446, -6.8819)
  line L378 (126.446, -6.8819) -> (125.645, -6.8819)
  line L379 (125.645, -6.8819) -> (125.645, -3.7827)
  line L380 (125.645, -3.7827) -> (126.446, -3.7827)
  line L381 (126.446, -3.7827) -> (126.446, -1.7823)
  line L382 (83.2954, -1.7823) -> (83.2954, -3.7827)
  line L383 (83.2954, -3.7827) -> (84.0962, -3.7827)
  line L384 (84.0962, -3.7827) -> (84.0962, -6.8819)
  line L385 (84.0962, -6.8819) -> (83.2954, -6.8819)
  line L386 (83.2954, -6.8819) -> (83.2954, -12.6821)
  line L387 (83.2954, -12.6821) -> (84.0962, -12.6821)
  line L388 (84.0962, -12.6821) -> (84.0962, -15.7827)
  line L389 (84.0962, -15.7827) -> (83.2954, -15.7827)
  line L390 (83.2954, -15.7827) -> (83.2954, -17.7817)
  line L391 (69.2961, -17.7817) -> (69.2961, -15.7827)
  line L392 (69.2961, -15.7827) -> (68.4953, -15.7827)
  line L393 (68.4953, -15.7827) -> (68.4953, -12.6821)
  line L394 (68.4953, -12.6821) -> (69.2961, -12.6821)
  line L395 (69.2961, -12.6821) -> (69.2961, -6.8819)
  line L396 (69.2961, -6.8819) -> (68.4953, -6.8819)
  line L397 (68.4953, -6.8819) -> (68.4953, -3.7827)
  line L398 (68.4953, -3.7827) -> (69.2961, -3.7827)
  line L399 (69.2961, -3.7827) -> (69.2961, -1.7823)
  line L400 (64.2454, -15.7827) -> (64.2454, -17.7817)
  line L401 (50.2461, -17.7817) -> (50.2461, -15.7827)
  line L402 (50.2461, -15.7827) -> (49.4453, -15.7827)
  line L403 (49.4453, -15.7827) -> (49.4453, -12.6821)
  line L404 (49.4453, -12.6821) -> (50.2461, -12.6821)
  line L405 (50.2461, -12.6821) -> (50.2461, -6.8819)
  line L406 (50.2461, -6.8819) -> (49.4453, -6.8819)
  line L407 (49.4453, -6.8819) -> (49.4453, -3.7827)
  line L408 (49.4453, -3.7827) -> (50.2461, -3.7827)
  line L409 (50.2461, -3.7827) -> (50.2461, -1.7823)
  line L410 (64.2454, -1.7823) -> (64.2454, -3.7827)
  line L411 (64.2454, -3.7827) -> (65.0462, -3.7827)
  line L412 (65.0462, -3.7827) -> (65.0462, -6.8819)
  line L413 (65.0462, -6.8819) -> (64.2454, -6.8819)
  line L414 (64.2454, -6.8819) -> (64.2454, -12.6821)
  line L415 (64.2454, -12.6821) -> (65.0462, -12.6821)
  line L416 (65.0462, -12.6821) -> (65.0462, -15.7827)
  line L417 (65.0462, -15.7827) -> (64.2454, -15.7827)
  line L418 (45.9962, -6.8819) -> (45.1954, -6.8819)
  line L419 (45.1954, -6.8819) -> (45.1954, -12.6821)
  line L420 (45.1954, -12.6821) -> (45.9962, -12.6821)
  line L421 (45.9962, -12.6821) -> (45.9962, -15.7827)
  line L422 (45.9962, -15.7827) -> (45.1954, -15.7827)
  line L423 (45.1954, -15.7827) -> (45.1954, -17.7817)
  line L424 (31.196, -17.7817) -> (31.196, -15.7827)
  line L425 (31.196, -15.7827) -> (30.3954, -15.7827)
  line L426 (30.3954, -15.7827) -> (30.3954, -12.6821)
  line L427 (30.3954, -12.6821) -> (31.196, -12.6821)
  line L428 (31.196, -12.6821) -> (31.196, -6.8819)
  line L429 (31.196, -6.8819) -> (30.3954, -6.8819)
  line L430 (30.3954, -6.8819) -> (30.3954, -3.7827)
  line L431 (30.3954, -3.7827) -> (31.196, -3.7827)
  line L432 (31.196, -3.7827) -> (31.196, -1.7823)
  line L433 (45.1954, -1.7823) -> (45.1954, -3.7827)
  line L434 (45.1954, -3.7827) -> (45.9962, -3.7827)
  line L435 (45.9962, -3.7827) -> (45.9962, -6.8819)
  line L436 (160.296, -6.8819) -> (159.495, -6.8819)
  line L437 (159.495, -6.8819) -> (159.495, -12.6821)
  line L438 (159.495, -12.6821) -> (160.296, -12.6821)
  line L439 (160.296, -12.6821) -> (160.296, -15.7827)
  line L440 (160.296, -15.7827) -> (159.495, -15.7827)
  line L441 (159.495, -15.7827) -> (159.495, -17.7817)
  line L442 (145.496, -17.7817) -> (145.496, -15.7827)
  line L443 (145.496, -15.7827) -> (144.695, -15.7827)
  line L444 (144.695, -15.7827) -> (144.695, -12.6821)
  line L445 (144.695, -12.6821) -> (145.496, -12.6821)
  line L446 (145.496, -12.6821) -> (145.496, -6.8819)
  line L447 (145.496, -6.8819) -> (144.695, -6.8819)
  line L448 (144.695, -6.8819) -> (144.695, -3.7827)
  line L449 (144.695, -3.7827) -> (145.496, -3.7827)
  line L450 (145.496, -3.7827) -> (145.496, -1.7823)
  line L451 (159.495, -1.7823) -> (159.495, -3.7827)
  line L452 (159.495, -3.7827) -> (160.296, -3.7827)
  line L453 (160.296, -3.7827) -> (160.296, -6.8819)
  line L454 (11.3454, -12.6821) -> (12.146, -12.6821)
  line L455 (12.146, -12.6821) -> (12.146, -6.8819)
  line L456 (12.146, -6.8819) -> (11.3454, -6.8819)
  line L457 (11.3454, -6.8819) -> (11.3454, -3.7827)
  line L458 (11.3454, -3.7827) -> (12.146, -3.7827)
  line L459 (12.146, -3.7827) -> (12.146, -1.7823)
  line L460 (26.1455, -1.7823) -> (26.1455, -3.7827)
  line L461 (26.1455, -3.7827) -> (26.9462, -3.7827)
  line L462 (26.9462, -3.7827) -> (26.9462, -6.8819)
  line L463 (26.9462, -6.8819) -> (26.1455, -6.8819)
  line L464 (26.1455, -6.8819) -> (26.1455, -12.6821)
  line L465 (26.1455, -12.6821) -> (26.9462, -12.6821)
  line L466 (26.9462, -12.6821) -> (26.9462, -15.7827)
  line L467 (26.9462, -15.7827) -> (26.1455, -15.7827)
  line L468 (26.1455, -15.7827) -> (26.1455, -17.7817)
  line L469 (12.146, -17.7817) -> (12.146, -15.7827)
  line L470 (12.146, -15.7827) -> (11.3454, -15.7827)
  line L471 (11.3454, -15.7827) -> (11.3454, -12.6821)
  line L472 (116.92, -25.9319) -> (116.119, -25.9319)
  line L473 (116.119, -25.9319) -> (116.119, -22.8327)
  line L474 (116.119, -22.8327) -> (116.92, -22.8327)
  line L475 (116.92, -22.8327) -> (116.92, -20.8323)
  line L476 (130.92, -20.8323) -> (130.92, -22.8327)
  line L477 (130.92, -22.8327) -> (131.721, -22.8327)
  line L478 (131.721, -22.8327) -> (131.721, -25.9319)
  line L479 (131.721, -25.9319) -> (130.92, -25.9319)
  line L480 (130.92, -25.9319) -> (130.92, -31.7321)
  line L481 (130.92, -31.7321) -> (131.721, -31.7321)
  line L482 (131.721, -31.7321) -> (131.721, -34.8327)
  line L483 (131.721, -34.8327) -> (130.92, -34.8327)
  line L484 (130.92, -34.8327) -> (130.92, -36.8316)
  line L485 (116.92, -36.8316) -> (116.92, -34.8327)
  line L486 (116.92, -34.8327) -> (116.119, -34.8327)
  line L487 (116.119, -34.8327) -> (116.119, -31.7321)
  line L488 (116.119, -31.7321) -> (116.92, -31.7321)
  line L489 (116.92, -31.7321) -> (116.92, -25.9319)
  line L490 (169.02, -25.9319) -> (169.02, -31.7321)
  line L491 (169.02, -31.7321) -> (169.821, -31.7321)
  line L492 (169.821, -31.7321) -> (169.821, -34.8327)
  line L493 (169.821, -34.8327) -> (169.02, -34.8327)
  line L494 (169.02, -34.8327) -> (169.02, -36.8316)
  line L495 (155.021, -36.8316) -> (155.021, -34.8327)
  line L496 (155.021, -34.8327) -> (154.22, -34.8327)
  line L497 (154.22, -34.8327) -> (154.22, -31.7321)
  line L498 (154.22, -31.7321) -> (155.021, -31.7321)
  line L499 (155.021, -31.7321) -> (155.021, -25.9319)
  line L500 (155.021, -25.9319) -> (154.22, -25.9319)
  line L501 (154.22, -25.9319) -> (154.22, -22.8327)
  line L502 (154.22, -22.8327) -> (155.021, -22.8327)
  line L503 (155.021, -22.8327) -> (155.021, -20.8323)
  line L504 (169.02, -20.8323) -> (169.02, -22.8327)
  line L505 (169.02, -22.8327) -> (169.821, -22.8327)
  line L506 (169.821, -22.8327) -> (169.821, -25.9319)
  line L507 (169.821, -25.9319) -> (169.02, -25.9319)
  line L508 (135.971, -34.8327) -> (135.17, -34.8327)
  line L509 (135.17, -34.8327) -> (135.17, -31.7321)
  line L510 (135.17, -31.7321) -> (135.971, -31.7321)
  line L511 (135.971, -31.7321) -> (135.971, -25.9319)
  line L512 (135.971, -25.9319) -> (135.17, -25.9319)
  line L513 (135.17, -25.9319) -> (135.17, -22.8327)
  line L514 (135.17, -22.8327) -> (135.971, -22.8327)
  line L515 (135.971, -22.8327) -> (135.971, -20.8323)
  line L516 (149.97, -20.8323) -> (149.97, -22.8327)
  line L517 (149.97, -22.8327) -> (150.771, -22.8327)
  line L518 (150.771, -22.8327) -> (150.771, -25.9319)
  line L519 (150.771, -25.9319) -> (149.97, -25.9319)
  line L520 (149.97, -25.9319) -> (149.97, -31.7321)
  line L521 (149.97, -31.7321) -> (150.771, -31.7321)
  line L522 (150.771, -31.7321) -> (150.771, -34.8327)
  line L523 (150.771, -34.8327) -> (149.97, -34.8327)
  line L524 (149.97, -34.8327) -> (149.97, -36.8316)
  line L525 (135.971, -36.8316) -> (135.971, -34.8327)
  line L526 (174.071, -25.9319) -> (173.27, -25.9319)
  line L527 (173.27, -25.9319) -> (173.27, -22.8327)
  line L528 (173.27, -22.8327) -> (174.071, -22.8327)
  line L529 (174.071, -22.8327) -> (174.071, -20.8323)
  line L530 (188.07, -20.8323) -> (188.07, -22.8327)
  line L531 (188.07, -22.8327) -> (188.871, -22.8327)
  line L532 (188.871, -22.8327) -> (188.871, -25.9319)
  line L533 (188.871, -25.9319) -> (188.07, -25.9319)
  line L534 (188.07, -25.9319) -> (188.07, -31.7321)
  line L535 (188.07, -31.7321) -> (188.871, -31.7321)
  line L536 (188.871, -31.7321) -> (188.871, -34.8327)
  line L537 (188.871, -34.8327) -> (188.07, -34.8327)
  line L538 (188.07, -34.8327) -> (188.07, -36.8316)
  line L539 (174.071, -36.8316) -> (174.071, -34.8327)
  line L540 (174.071, -34.8327) -> (173.27, -34.8327)
  line L541 (173.27, -34.8327) -> (173.27, -31.7321)
  line L542 (173.27, -31.7321) -> (174.071, -31.7321)
  line L543 (174.071, -31.7321) -> (174.071, -25.9319)
  line L544 (0.0951, -55.4069) -> (0.102, -55.5639)
  line L545 (0.102, -55.5639) -> (0.1199, -55.7209)
  line L546 (0.1199, -55.7209) -> (0.1502, -55.874)
  line L547 (0.1502, -55.874) -> (0.1929, -56.0268)
  line L548 (0.1929, -56.0268) -> (0.248, -56.1728)
  line L549 (0.248, -56.1728) -> (0.3128, -56.315)
  line L550 (0.3128, -56.315) -> (0.39, -56.4526)
  line L551 (0.39, -56.4526) -> (0.4768, -56.5838)
  line L552 (0.4768, -56.5838) -> (0.5746, -56.7062)
  line L553 (0.5746, -56.7062) -> (0.6808, -56.8219)
  line L554 (0.6808, -56.8219) -> (0.7965, -56.9281)
  line L555 (0.7965, -56.9281) -> (0.9192, -57.0258)
  line L556 (0.9192, -57.0258) -> (1.0501, -57.113)
  line L557 (1.0501, -57.113) -> (1.1879, -57.1899)
  line L558 (1.1879, -57.1899) -> (1.3298, -57.2548)
  line L559 (1.3298, -57.2548) -> (1.4759, -57.3098)
  line L560 (1.4759, -57.3098) -> (1.6288, -57.3525)
  line L561 (1.6288, -57.3525) -> (1.7818, -57.3828)
  line L562 (1.7818, -57.3828) -> (1.9389, -57.4008)
  line L563 (1.9389, -57.4008) -> (2.096, -57.4075)
  line L564 (2.096, -57.4075) -> (6.5216, -57.4075)
  line L565 (188.597, -57.4075) -> (188.753, -57.4008)
  line L566 (188.753, -57.4008) -> (188.908, -57.3828)
  line L567 (188.908, -57.3828) -> (189.063, -57.3525)
  line L568 (189.063, -57.3525) -> (189.214, -57.3098)
  line L569 (189.214, -57.3098) -> (189.362, -57.2548)
  line L570 (189.362, -57.2548) -> (189.504, -57.1899)
  line L571 (189.504, -57.1899) -> (189.64, -57.113)
  line L572 (189.64, -57.113) -> (189.771, -57.0258)
  line L573 (189.771, -57.0258) -> (189.895, -56.9281)
  line L574 (189.895, -56.9281) -> (190.011, -56.8219)
  line L575 (190.011, -56.8219) -> (190.117, -56.7062)
  line L576 (190.117, -56.7062) -> (190.215, -56.5838)
  line L577 (190.215, -56.5838) -> (190.302, -56.4526)
  line L578 (190.302, -56.4526) -> (190.379, -56.315)
  line L579 (190.379, -56.315) -> (190.444, -56.1728)
  line L580 (190.444, -56.1728) -> (190.499, -56.0268)
  line L581 (190.499, -56.0268) -> (190.54, -55.874)
  line L582 (190.54, -55.874) -> (190.572, -55.7209)
  line L583 (190.572, -55.7209) -> (190.59, -55.5639)
  line L584 (190.59, -55.5639) -> (190.596, -55.4069)
  line L585 (190.596, -55.4069) -> (190.596, -2.2572)
  line L586 (190.596, -2.2572) -> (190.59, -2.1001)
  line L587 (190.59, -2.1001) -> (190.572, -1.9444)
  line L588 (190.572, -1.9444) -> (190.54, -1.7901)
  line L589 (190.54, -1.7901) -> (190.499, -1.6385)
  line L590 (190.499, -1.6385) -> (190.444, -1.491)
  line L591 (190.444, -1.491) -> (190.379, -1.3491)
  line L592 (190.379, -1.3491) -> (190.302, -1.2127)
  line L593 (190.302, -1.2127) -> (190.215, -1.0818)
  line L594 (190.215, -1.0818) -> (190.117, -0.9577)
  line L595 (190.117, -0.9577) -> (190.011, -0.842)
  line L596 (190.011, -0.842) -> (189.895, -0.7359)
  line L597 (189.895, -0.7359) -> (189.771, -0.638)
  line L598 (189.771, -0.638) -> (189.64, -0.5512)
  line L599 (189.64, -0.5512) -> (189.504, -0.474)
  line L600 (189.504, -0.474) -> (189.362, -0.4093)
  line L601 (189.362, -0.4093) -> (189.214, -0.3542)
  line L602 (189.214, -0.3542) -> (189.063, -0.3128)
  line L603 (189.063, -0.3128) -> (188.908, -0.2811)
  line L604 (188.908, -0.2811) -> (188.753, -0.2632)
  line L605 (188.753, -0.2632) -> (188.597, -0.2563)
  line L606 (188.597, -0.2563) -> (167.0351, -0.2565)
  line L607 (2.096, -0.2577) -> (1.9389, -0.2632)
  line L608 (1.9389, -0.2632) -> (1.7818, -0.2811)
  line L609 (1.7818, -0.2811) -> (1.6288, -0.3128)
  line L610 (1.6288, -0.3128) -> (1.4759, -0.3542)
  line L611 (1.4759, -0.3542) -> (1.3298, -0.4093)
  line L612 (1.3298, -0.4093) -> (1.1879, -0.474)
  line L613 (1.1879, -0.474) -> (1.0501, -0.5512)
  line L614 (1.0501, -0.5512) -> (0.9192, -0.638)
  line L615 (0.9192, -0.638) -> (0.7965, -0.7359)
  line L616 (0.7965, -0.7359) -> (0.6808, -0.842)
  line L617 (0.6808, -0.842) -> (0.5746, -0.9577)
  line L618 (0.5746, -0.9577) -> (0.4768, -1.0818)
  line L619 (0.4768, -1.0818) -> (0.39, -1.2127)
  line L620 (0.39, -1.2127) -> (0.3128, -1.3491)
  line L621 (0.3128, -1.3491) -> (0.248, -1.491)
  line L622 (0.248, -1.491) -> (0.1929, -1.6385)
  line L623 (0.1929, -1.6385) -> (0.1502, -1.7901)
  line L624 (0.1502, -1.7901) -> (0.1199, -1.9444)
  line L625 (0.1199, -1.9444) -> (0.102, -2.1001)
  line L626 (0.102, -2.1001) -> (0.0951, -2.2572)
  line L627 (0.0951, -2.2572) -> (0.0951, -55.4069)
  line L628 (182.846, -0.0227) -> (190.596, -0.0227)
  line L629 (190.596, -0.0227) -> (190.596, -16.7817)
  line L630 (190.596, -16.7817) -> (182.846, -16.7817)
  line L631 (182.846, -16.7817) -> (182.846, -0.0227)
  line L632 (0.0951, -16.7817) -> (7.8454, -16.7817)
  line L633 (7.8454, -16.7817) -> (7.8454, -0.2577)
  line L634 (7.8454, -0.2577) -> (0.0951, -0.2576)
  line L635 (0.0951, -0.2576) -> (0.0951, -16.7817)
  line L636 (159.495, -17.7817) -> (145.496, -17.7817)
  line L637 (145.496, -1.7823) -> (159.495, -1.7823)
  line L638 (31.196, -1.7823) -> (45.1954, -1.7823)
  line L639 (45.1954, -17.7817) -> (31.196, -17.7817)
  line L640 (155.021, -20.8323) -> (169.02, -20.8323)
  line L641 (169.02, -36.8316) -> (155.021, -36.8316)
  line L642 (135.971, -20.8323) -> (149.97, -20.8323)
  line L643 (149.97, -36.8316) -> (135.971, -36.8316)
  line L644 (116.92, -20.8323) -> (130.92, -20.8323)
  line L645 (130.92, -36.8316) -> (116.92, -36.8316)
  line L646 (111.869, -36.8316) -> (97.8697, -36.8316)
  line L647 (97.8697, -20.8323) -> (111.869, -20.8323)
  line L648 (40.7211, -20.8323) -> (54.7204, -20.8323)
  line L649 (54.7204, -36.8316) -> (40.7211, -36.8316)
  line L650 (35.6704, -36.8316) -> (21.671, -36.8316)
  line L651 (21.671, -20.8323) -> (35.6704, -20.8323)
  line L652 (155.021, -39.8824) -> (169.02, -39.8824)
  line L653 (169.02, -55.8816) -> (155.021, -55.8816)
  line L654 (16.6205, -36.8316) -> (2.621, -36.8316)
  line L655 (2.621, -20.8323) -> (16.6205, -20.8323)
  line L656 (21.671, -39.8824) -> (35.6704, -39.8824)
  line L657 (35.6704, -55.8816) -> (21.671, -55.8816)
  line L658 (97.8697, -39.8824) -> (111.869, -39.8824)
  line L659 (111.869, -55.8816) -> (97.8697, -55.8816)
  line L660 (54.7204, -55.8816) -> (40.7211, -55.8816)
  line L661 (40.7211, -39.8824) -> (54.7204, -39.8824)
  line L662 (92.8204, -36.8316) -> (78.8211, -36.8316)
  line L663 (78.8211, -20.8323) -> (92.8204, -20.8323)
  line L664 (130.92, -55.8816) -> (116.92, -55.8816)
  line L665 (116.92, -39.8824) -> (130.92, -39.8824)
  line L666 (188.07, -36.8316) -> (174.071, -36.8316)
  line L667 (174.071, -20.8323) -> (188.07, -20.8323)
  line L668 (69.2961, -1.7823) -> (83.2954, -1.7823)
  line L669 (83.2954, -17.7817) -> (69.2961, -17.7817)
  line L670 (164.546, -1.7823) -> (178.545, -1.7823)
  line L671 (178.545, -17.7817) -> (164.546, -17.7817)
  line L672 (64.2454, -17.7817) -> (50.2461, -17.7817)
  line L673 (50.2461, -1.7823) -> (64.2454, -1.7823)
  line L674 (126.446, -1.7823) -> (140.445, -1.7823)
  line L675 (140.445, -17.7817) -> (126.446, -17.7817)
  line L676 (92.8204, -55.8816) -> (78.8211, -55.8816)
  line L677 (78.8211, -39.8824) -> (92.8204, -39.8824)
  line L678 (135.971, -39.8824) -> (149.97, -39.8824)
  line L679 (149.97, -55.8816) -> (135.971, -55.8816)
  line L680 (59.7711, -39.8824) -> (73.7704, -39.8824)
  line L681 (73.7704, -55.8816) -> (59.7711, -55.8816)
  line L682 (16.6205, -55.8816) -> (2.621, -55.8816)
  line L683 (2.621, -39.8824) -> (16.6205, -39.8824)
  line L684 (174.071, -39.8824) -> (188.07, -39.8824)
  line L685 (188.07, -55.8816) -> (174.071, -55.8816)
  line L686 (73.7704, -36.8316) -> (59.7711, -36.8316)
  line L687 (59.7711, -20.8323) -> (73.7704, -20.8323)
  line L688 (26.1455, -17.7817) -> (12.146, -17.7817)
  line L689 (12.146, -1.7823) -> (26.1455, -1.7823)
  line L690 (111.87, -17.7817) -> (97.8711, -17.7817)
  line L691 (97.8711, -1.7823) -> (111.87, -1.7823)
  line L692 (6.5216, -57.4075) -> (35.7006, -57.4075)
  line L693 (35.7006, -57.4075) -> (154.9924, -57.4075)
  line L694 (154.9924, -57.4075) -> (184.1714, -57.4075)
  line L695 (184.1714, -57.4075) -> (188.597, -57.4075)
  line L696 (167.0351, -0.2565) -> (137.8078, -0.2567)
  line L697 (137.8078, -0.2567) -> (52.887, -0.2573)
  line L698 (52.887, -0.2573) -> (23.4739, -0.2575)
  line L699 (23.4739, -0.2575) -> (2.096, -0.2577)
  dimension "d29" = 3.5
  dimension "d32" = 3.5
  constraint horizontal L628
  constraint vertical L629
  constraint horizontal L630
  constraint vertical L631
  constraint coincident L585 L629.end
  constraint horizontal L632
  constraint vertical L633
  constraint horizontal L634
  constraint vertical L635
  constraint coincident L627 L632.start
  measures "d29" distance of L297 L631
  measures "d32" distance of L471 L633
extrude "Extrude5" cut sketch "Sketch4" against normal blind 55 contours L607 L608 L609 L610 L611 L612 L613 L614 L615 L616 L617 L618 L619 L620 L621 L622 L623 L624 L625 L626 L627 L632 L633 L634 L635 L699 | L585 L586 L587 L588 L589 L590 L591 L592 L593 L594 L595 L596 L597 L598 L599 L600 L601 L602 L603 L604 L605 L606 L629 L630 L631
fillet "Fillet1" radius 2 3 edges at (0.0951, -2, -16.7817) (7.8454, -2, -16.7817) (7.8454, -2, -0.2577)
fillet "Fillet1" radius 2 3 edges at (182.846, -2, -16.7817) (182.846, -2, -0.2564) (190.596, -2, -16.7817)